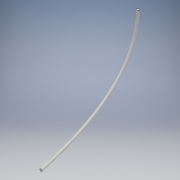
# Autodesk Inventor part: Rib
Saved by Autodesk Inventor 2018 (Build 220112000, 112)
## iProperties
Created: 2019-06-02
Part Number: Rib
Material: Generic
Document SubType Name: Modeling
Designer: dell
Density: 1 g/cm^3
Appearance: Default
Author: dell
Autodesk Inventor part; units mm, degrees
ref_plane "YZ Plane" through (0, 0, 0) normal (1, 0, 0) x (0, 1, 0)
ref_plane "XZ Plane" through (0, 0, 0) normal (0, 1, 0) x (-1, 0, 0)
sketch "Sketch1" plane through (0, 0, 0) normal (1, 0, 0) x (0, 1, 0)
  spline S0 degree 2 poles (800, 0) (798.6366, -529.7903) (0, -750) knots 0 0 0 1 1 1
  point P0 (0, 0)
  point P1 (650, -400)
  dimension "d1" = 750
  dimension "d3" = 400
  dimension "d4" = 150
  dimension "d5" = 350
  constraints: 3 other
  measures "d1" distance of point (0, -750) point (0, 0)
  measures "d3" vertical distance of point (800, 0) point (650, -400)
  measures "d4" horizontal distance of point (800, 0) point (650, -400)
  measures "d5" vertical distance of point (650, -400) point (0, -750)
sketch "Sketch3" plane through (0, 0, 0) normal (0, 1, 0) x (-1, 0, 0)
  circle A0 centre (0, -750) radius 10
  point P0 (0, 0)
  dimension "d6" = 20
  constraints: 1 centre point, 1 coincident
  measures "d6" diameter of A0
sweep "Sweep1" add profiles "Sketch3" path "Sketch1"
sketch "Sketch4" plane through (0, 0, 0) normal (1, 0, 0) x (0, 1, 0)
  circle A0 centre (799.6334, -5.0882) radius 1
  line L0 (809.6334, -2.6829) -> (790.3666, 2.6829) projected
  point P0 (0, 0)
  point P1 (800, 0)
  dimension "d9" = 2
  dimension "d10" = 5
  dimension "d12" = 10
  constraints: 1 centre point
  measures "d9" diameter of A0
  measures "d10" distance from line of L0 A0.centre
  measures "d12" horizontal distance of L0.start A0.centre
extrude "Extrusion1" cut sketch "Sketch4" along normal mid plane 20
ref_plane "Work Plane1" through (0, 0, 3) normal (0, 0, 1) x (1, 0, 0)
body "Solid1"
